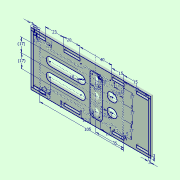
# Autodesk Inventor part: Bottom_plate2
Saved by Autodesk Inventor 2015 (Build 190159000, 159)
## iProperties
Created: 2015-06-18
Part Number: Bottom_plate2
Material: Generic
Document SubType Name: Modeling
Designer: Openlab
Density: 1 g/cm^3
Appearance: Polycarbonate - Clear
Author: Openlab
Autodesk Inventor part; units mm, degrees
ref_plane "YZ Plane" through (0, 0, 0) normal (1, 0, 0) x (0, 1, 0)
ref_plane "XZ Plane" through (0, 0, 0) normal (0, 1, 0) x (-1, 0, 0)
ref_plane "XY Plane" through (0, 0, 0) normal (0, 0, 1) x (1, 0, 0)
sketch "Sketch1" plane through (0, 0, 0) normal (0, 1, 0) x (-1, 0, 0)
  line L0 (41.25, -2.25) -> (28.75, -2.25) construction
  line L1 (28.75, -2.25) -> (28.75, -14.75) construction
  line L2 (28.75, -14.75) -> (41.25, -14.75) construction
  line L3 (41.25, -14.75) -> (41.25, -2.25) construction
  line L4 (56.9183, -8.5) -> (8.3915, -8.5) construction
  line L5 (0, -17) -> (105, -17) construction
  line L6 (0, 0) -> (0, -51) construction
  line L7 (0, -34) -> (105, -34) construction
  line L8 (105, -51) -> (105, 0) construction
  line L9 (35, 19) -> (35, -51) construction
  line L10 (56.8064, -25.5) -> (17, -25.5) construction
  line L11 (28.75, -19.25) -> (28.75, -31.75) construction
  line L12 (41.25, -19.25) -> (28.75, -19.25) construction
  line L13 (41.25, -31.75) -> (41.25, -19.25) construction
  line L14 (28.75, -31.75) -> (41.25, -31.75) construction
  line L15 (28.75, -36.25) -> (28.75, -48.75) construction
  line L16 (41.25, -36.25) -> (28.75, -36.25) construction
  line L17 (41.25, -48.75) -> (41.25, -36.25) construction
  line L18 (28.75, -48.75) -> (41.25, -48.75) construction
  line L19 (56.3008, -42.5) -> (16.5498, -42.5) construction
  arc A0 (53.45, -12) -> (53.45, -22) centre (53.45, -17) ccw
  arc A1 (92, -22) -> (92, -12) centre (92, -17) ccw
  arc A2 (53.45, -29) -> (53.45, -39) centre (53.45, -34) ccw
  arc A3 (92, -39) -> (92, -29) centre (92, -34) ccw
  line L20 (53.45, -12) -> (92, -12)
  line L21 (53.45, -22) -> (92, -22)
  line L22 (53.45, -29) -> (92, -29)
  line L23 (53.45, -39) -> (92, -39)
  arc A4 (16.15, -39) -> (16.15, -29) centre (16.15, -34) ccw
  line L24 (103.5, -49.5) -> (103.5, -1.5) construction
  line L25 (1.5, -1.5) -> (1.5, -49.5) construction
  arc A5 (14, -29) -> (14, -39) centre (14, -34) ccw
  arc A6 (14, -12) -> (14, -22) centre (14, -17) ccw
  line L26 (16.15, -39) -> (14, -39)
  line L27 (14, -29) -> (16.15, -29)
  line L28 (14, -22) -> (16.15, -22)
  line L29 (16.15, -12) -> (14, -12)
  arc A7 (16.15, -22) -> (16.15, -12) centre (16.15, -17) ccw
  arc A8 (96.5, -51) -> (93, -47.5) centre (93, -51) ccw construction
  arc A9 (53.45, -47.5) -> (49.95, -51) centre (53.45, -51) ccw construction
  arc A10 (97.7697, -49.5) -> (93, -46) centre (93, -51) ccw construction
  line L30 (93, -46) -> (53.45, -46) construction
  line L31 (96.5, -51) -> (105, -51) construction
  line L32 (93, -47.5) -> (53.45, -47.5) construction
  line L33 (105, -49.5) -> (97.7697, -49.5) construction
  arc A11 (53.45, -46) -> (48.6803, -49.5) centre (53.45, -51) ccw construction
  arc A12 (48.6803, -1.5) -> (53.45, -5) centre (53.45, 0) ccw construction
  arc A13 (49.95, 0) -> (53.45, -3.5) centre (53.45, 0) ccw construction
  line L34 (93, -3.5) -> (53.45, -3.5) construction
  line L35 (93, -5) -> (53.45, -5) construction
  line L36 (97.7697, -1.5) -> (105, -1.5) construction
  line L37 (105, 0) -> (96.5, 0) construction
  arc A14 (93, -3.5) -> (96.5, 0) centre (93, 0) ccw construction
  arc A15 (93, -5) -> (97.7697, -1.5) centre (93, 0) ccw construction
  arc A16 (20.65, -51) -> (17.15, -47.5) centre (17.15, -51) ccw construction
  arc A17 (12, -47.5) -> (8.5, -51) centre (12, -51) ccw construction
  line L38 (17.15, -46) -> (12, -46) construction
  line L39 (17.15, -47.5) -> (12, -47.5) construction
  arc A18 (12, -46) -> (7.2303, -49.5) centre (12, -51) ccw construction
  arc A19 (21.9197, -49.5) -> (17.15, -46) centre (17.15, -51) ccw construction
  line L40 (48.6803, -49.5) -> (21.9197, -49.5) construction
  line L41 (7.2303, -49.5) -> (0, -49.5) construction
  line L42 (0, -51) -> (8.5, -51) construction
  line L43 (20.65, -51) -> (49.95, -51) construction
  line L44 (17.15, -5) -> (12, -5) construction
  line L45 (17.15, -3.5) -> (12, -3.5) construction
  arc A20 (8.5, 0) -> (12, -3.5) centre (12, 0) ccw construction
  arc A21 (17.15, -3.5) -> (20.65, 0) centre (17.15, 0) ccw construction
  arc A22 (7.2303, -1.5) -> (12, -5) centre (12, 0) ccw construction
  arc A23 (17.15, -5) -> (21.9197, -1.5) centre (17.15, 0) ccw construction
  line L46 (49.95, 0) -> (20.65, 0) construction
  line L47 (8.5, 0) -> (0, 0) construction
  line L48 (0, -1.5) -> (7.2303, -1.5) construction
  line L49 (21.9197, -1.5) -> (48.6803, -1.5) construction
  line L50 (-30, 2) -> (-30, -53)
  line L51 (113, -53) -> (113, 2)
  arc A24 (42.75, -4.25) -> (39.25, -0.75) centre (39.25, -4.25) ccw
  arc A25 (30.75, -0.75) -> (27.25, -4.25) centre (30.75, -4.25) ccw
  arc A26 (39.25, -50.25) -> (42.75, -46.75) centre (39.25, -46.75) ccw
  arc A27 (27.25, -46.75) -> (30.75, -50.25) centre (30.75, -46.75) ccw
  line L52 (42.75, -4.25) -> (42.75, -46.75)
  line L53 (39.25, -0.75) -> (30.75, -0.75)
  line L54 (27.25, -4.25) -> (27.25, -46.75)
  line L55 (30.75, -50.25) -> (39.25, -50.25)
  line L56 (113, 2) -> (113, 5)
  line L57 (-30, 5) -> (-30, 2)
  line L58 (113, -53) -> (113, -56)
  line L59 (-30, -56) -> (-30, -53)
  line L60 (113, 5) -> (116, 5)
  line L61 (116, 5) -> (116, -56)
  line L62 (116, -56) -> (113, -56)
  line L63 (-30, -56) -> (-33, -56)
  line L64 (-33, -56) -> (-33, 5)
  line L65 (-33, 5) -> (-30, 5)
  line L66 (55, 5) -> (55, 2)
  line L67 (75, 5) -> (75, 2)
  line L68 (98, 5) -> (98, 2)
  line L69 (15, 5) -> (15, 2)
  line L70 (0, 2) -> (0, 5)
  line L71 (55, -56) -> (55, -53)
  line L72 (15, -56) -> (15, -53)
  line L73 (0, -56) -> (0, -53)
  line L74 (75, -56) -> (75, -53)
  line L75 (98, -56) -> (98, -53)
  line L76 (-15, 5) -> (-15, 2)
  line L77 (-15, -53) -> (-15, -56)
  line L78 (116, 5) -> (116, 8)
  line L79 (116, 8) -> (-33, 8)
  line L80 (-33, 8) -> (-33, 5)
  line L81 (-33, -56) -> (-33, -59)
  line L82 (-33, -59) -> (116, -59)
  line L83 (116, -59) -> (116, -56)
  line L84 (15, 5) -> (0, 5)
  line L85 (15, 2) -> (0, 2)
  line L86 (113, 5) -> (98, 5)
  line L87 (75, 5) -> (55, 5)
  line L88 (113, 2) -> (98, 2)
  line L89 (75, 2) -> (55, 2)
  line L90 (55, -53) -> (75, -53)
  line L91 (98, -53) -> (113, -53)
  line L92 (113, -56) -> (98, -56)
  line L93 (75, -56) -> (55, -56)
  line L94 (-30, -53) -> (-15, -53)
  line L95 (0, -53) -> (15, -53)
  line L96 (15, -56) -> (0, -56)
  line L97 (-15, -56) -> (-30, -56)
  line L98 (-15, 2) -> (-30, 2)
  line L99 (-15, 5) -> (-30, 5)
  point P0 (35, -8.5)
  point P1 (35, -42.5)
  point P2 (35, -25.5)
  dimension "d0" = 12.5
  dimension "d1" = 12.5
  dimension "d2" = 17
  dimension "d3" = 35
  dimension "d4" = 105
  dimension "d5" = 17
  dimension "d6" = 17
  dimension "d7" = 10
  dimension "d8" = 1.5
  dimension "d9" = 1.5
  dimension "d10" = 5
  dimension "d11" = 1.5
  dimension "d12" = 1.5
  dimension "d13" = 1.5
  dimension "d14" = 17
  dimension "d15" = 17
  dimension "d16" = 12
  dimension "d17" = 13
  dimension "d18" = 12.2
  dimension "d19" = 11.6
  dimension "d20" = 12.6
  dimension "d21" = 12
  dimension "d22" = 12.5
  dimension "d24" = 8
  dimension "d25" = 30
  dimension "d28" = 2
  dimension "d29" = 2
  dimension "d30" = 7
  dimension "d31" = 2
  dimension "d32" = 2
  dimension "d40" = 3
  dimension "d42" = 3
  dimension "d43" = 3
  dimension "d44" = 40
  dimension "d45" = 15
  dimension "d46" = 15
  dimension "d47" = 20
  dimension "d48" = 23
  dimension "d49" = 3
  dimension "d50" = 3
  dimension "d51" = 3
  dimension "d52" = 2
  constraints: 200 end point, 82 perpendicular, 56 point on circle, 34 point on line, 32 tangent, 30 collinear, 28 centre point, 28 parallel, 24 equal radius, 16 horizontal, 11 vertical alignment, 10 coincident, 9 horizontal alignment, 3 vertical, 10 other
  measures "d0" distance of L2.end L1.end
  measures "d1" distance of L0.end L1.end
  measures "d2" distance between parallel lines of L10 L4
  measures "d3" distance between parallel lines of L6 L9
  measures "d4" distance between parallel lines of L6 L8
  measures "d5" distance between parallel lines of L19 L10
  measures "d6" distance between parallel lines of L5 L7
  measures "d7" diameter of A0
  measures "d8" distance between parallel lines of L6 L25
  measures "d9" distance between parallel lines of L8 L24
  measures "d10" radius of A4
  measures "d11" radial gap between concentric circles of A8 A10
  measures "d12" distance between parallel lines of L37 L36
  measures "d13" distance between parallel lines of L41 L42
  measures "d14" distance between parallel lines of L7 L42
  measures "d15" distance between parallel lines of L47 L5
  measures "d16" distance from line of A8.centre L8
  measures "d17" distance from line of L8 A3.centre
  measures "d18" distance from line of A9.centre L17
  measures "d19" distance from line of A19.centre L15
  measures "d20" distance from line of A4.centre L15
  measures "d21" distance from line of L6 A22.centre
  measures "d22" distance from line of L25 A6.centre
  measures "d24" distance between parallel lines of L8 L51
  measures "d25" distance between parallel lines of L50 L6
  measures "d28" distance from line of L1 A25.centre
  measures "d29" distance from line of A25.centre L0
  measures "d30" diameter of A25
  measures "d31" distance from line of L17 A26.centre
  measures "d32" distance from line of L18 A26.centre
  measures "d40" distance of L51.end L56.end
  measures "d42" distance of L56.end L60.end
  measures "d43" distance of L59.start L63.end
  measures "d44" distance between parallel lines of L69 L66
  measures "d45" distance between parallel lines of L70 L69
  measures "d46" distance between parallel lines of L76 L70
  measures "d47" distance between parallel lines of L67 L66
  measures "d48" distance between parallel lines of L68 L67
  measures "d49" distance of L60.end L78.end
  measures "d50" distance of L63.end L81.end
  measures "d51" distance between parallel lines of L93 L90
  measures "d52" distance between parallel lines of L88 L37
extrude "Extrusion2" add sketch "Sketch1" along normal blind 3 contours L98 L76 L99 L65 L80 L79 L78 L60 L86 L68 L88 L51 L91 L75 L92 L62 L83 L82 L81 L63 L97 L77 L94 L50 | L50 L59 L63 L64 L65 L57 | L61 L62 L58 L51 L56 L60 | L52 A26 L55 A27 L54 A25 L53 A24
hole "Hole1" at (-35, 0, -8.5) at (-35, 0, -42.5) at (-35, 0, -25.5) direction (0, 1, 0) diameter 8 end through all
body "Solid1"
